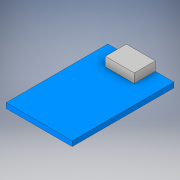
# Autodesk Inventor part: Wavgat_Battery_Charger
Saved by Autodesk Inventor 2019.4 (Build 234330000, 330)
## iProperties
Created: 2021-06-27
Part Number: Wavgat_Battery_Charger
Material: Generic
Document SubType Name: Modeling
Designer: keshav
Density: 1 g/cm^3
Appearance: Default
Author: keshav
Autodesk Inventor part; units mm, degrees
ref_plane "YZ Plane" through (0, 0, 0) normal (1, 0, 0) x (0, 1, 0)
ref_plane "XZ Plane" through (0, 0, 0) normal (0, 1, 0) x (-1, 0, 0)
ref_plane "XY Plane" through (0, 0, 0) normal (0, 0, 1) x (1, 0, 0)
sketch "Sketch1" plane through (0, 0, 0) normal (0, 1, 0) x (-1, 0, 0)
  line L0 (-8.5, 13.075) -> (8.5, 13.075)
  line L1 (8.5, 13.075) -> (8.5, -13.075)
  line L2 (8.5, -13.075) -> (-8.5, -13.075)
  line L3 (-8.5, -13.075) -> (-8.5, 13.075)
  line L4 (-8.5, 13.075) -> (8.5, -13.075) construction
  line L5 (8.5, 13.075) -> (-8.5, -13.075) construction
  point P0 (0, 0)
  dimension "d0" = 17
  dimension "d1" = 26.15
  constraints: 12 end point, 2 midpoint, 2 parallel, 1 horizontal, 1 perpendicular
  measures "d0" distance of L1.end L2.end
  measures "d1" distance of L0.end L1.end
extrude "Extrusion1" add sketch "Sketch1" along normal blind 1.3
sketch "Sketch3" plane through (0, 1.3, 0) normal (0, 1, 0) x (1, 0, 0)
  line L0 (8.5, 13.075) -> (-8.5, 13.075) construction
  line L1 (0, 13.075) -> (0, 0) construction
  line L2 (-3.725, 13.075) -> (-3.725, 7.65)
  line L3 (-3.725, 7.65) -> (0, 7.65)
  line L4 (-3.725, 13.075) -> (0, 13.075)
  line L5 (3.725, 13.075) -> (3.725, 7.65)
  line L6 (3.725, 7.65) -> (0, 7.65)
  line L7 (3.725, 13.075) -> (0, 13.075)
  dimension "d5" = 5.425
  dimension "d6" = 3.725
  constraints: 14 end point, 2 point on line, 2 symmetric about line, 2 vertical, 1 collinear, 1 midpoint, 1 perpendicular
  measures "d5" distance between parallel lines of L0 L3
  measures "d6" distance between parallel lines of L1 L2
extrude "Extrusion2" add sketch "Sketch3" along normal blind 2.35
body "Solid1"
